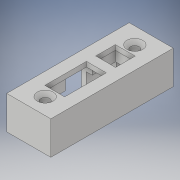
# Autodesk Inventor part: sharp1
Saved by Autodesk Inventor 2019 (Build 230136000, 136)
## iProperties
Created: 2019-04-30
Part Number: sharp1
Material: Générique
Document SubType Name: Modeling
Designer: dubicube
Density: 1 g/cm^3
Appearance: Par défaut
Author: dubicube
Autodesk Inventor part; units mm, degrees
ref_plane "YZ Plane" through (0, 0, 0) normal (1, 0, 0) x (0, 1, 0)
ref_plane "XZ Plane" through (0, 0, 0) normal (0, 1, 0) x (-1, 0, 0)
ref_plane "XY Plane" through (0, 0, 0) normal (0, 0, 1) x (1, 0, 0)
sketch "Esquisse1" plane through (0, 0, 0) normal (0, 1, 0) x (-1, 0, 0)
  line L0 (0, 0) -> (-18, 0)
  line L1 (-18, 0) -> (-18, -50)
  line L2 (-18, -50) -> (0, -50)
  line L3 (0, -50) -> (0, 0)
  dimension "d0" = 50
  dimension "d1" = 18
  constraints: 8 end point, 2 parallel, 1 coincident, 1 horizontal, 1 perpendicular
  measures "d0" distance of L2.end L0.start
  measures "d1" distance of L0.start L0.end
extrude "Extrusion1" add sketch "Esquisse1" along normal blind 13.6
sketch "Esquisse2" plane through (0, 0, 0) normal (0, -1, 0) x (1, 0, 0)
  line L0 (13.05, -10.6) -> (4.95, -10.6)
  line L1 (4.95, -10.6) -> (4.95, -27.6)
  line L2 (4.95, -39.4) -> (13.05, -39.4)
  line L3 (13.05, -39.4) -> (13.05, -31.4)
  line L4 (18, 0) -> (18, -50) projected
  line L5 (18, -25) -> (0, -25) construction
  line L6 (0, -50) -> (0, 0) projected
  line L7 (0, 0) -> (18, 0) projected
  line L8 (9, 0) -> (9, -50) construction
  line L9 (18, -50) -> (0, -50) projected
  line L10 (13.05, -31.4) -> (4.95, -31.4)
  line L11 (4.95, -27.6) -> (13.05, -27.6)
  line L12 (13.05, -31.4) -> (13.05, -27.6) construction
  line L13 (13.05, -27.6) -> (13.05, -10.6)
  line L14 (4.95, -27.6) -> (4.95, -31.4) construction
  line L15 (4.95, -31.4) -> (4.95, -39.4)
  point P0 (13.05, -25)
  point P1 (9, -10.6)
  dimension "d4" = 28.8
  dimension "d5" = 8.1
  dimension "d36" = 8
  dimension "d37" = 17
  constraints: 24 end point, 10 parallel, 9 perpendicular, 5 midpoint, 4 point on line, 1 horizontal
  measures "d4" distance of L2.end L0.start
  measures "d5" distance of L0.start L0.end
  measures "d36" distance between parallel lines of L2 L10
  measures "d37" distance between parallel lines of L0 L11
extrude "Extrusion2" cut sketch "Esquisse2" against normal blind 13.6 contours L13 L11 L1 L0 | L15 L10 L3 L2
sketch "Esquisse3" plane through (0, 0, 0) normal (0, -1, 0) x (1, 0, 0)
  circle A0 centre (9, -43.3) radius 1.75
  line L0 (4.95, -10.6) -> (13.05, -10.6) projected
  line L1 (0, -50) -> (0, 0) projected
  line L2 (18, -50) -> (0, -50) projected
  line L3 (9, -50) -> (9, 0)
  line L4 (0, 0) -> (18, 0) projected
  circle A1 centre (9, -6.7) radius 1.75
  line L5 (13.05, -39.4) -> (4.95, -39.4) projected
  dimension "d8" = 32.7
  dimension "d10" = 3.5
  dimension "d11" = 3.5
  dimension "d12" = 32.7
  constraints: 2 centre point, 2 end point, 2 midpoint, 2 point on line
  measures "d8" distance from line of A0.centre L0
  measures "d10" diameter of A0
  measures "d11" diameter of A1
  measures "d12" distance from line of A1.centre L5
extrude "Extrusion3" cut sketch "Esquisse3" against normal blind 13.6 contours A0 L3 | L3 A0 | A1 L3 | L3 A1
sketch "Esquisse4" plane through (0, 0, 0) normal (0, -1, 0) x (1, 0, 0)
  line L0 (13.55, -10) -> (13.55, -40)
  line L1 (13.55, -40) -> (4.45, -40)
  line L2 (4.45, -40) -> (4.45, -30.5)
  line L3 (4.45, -30.5) -> (0, -30.5)
  line L4 (0, -30.5) -> (0, -19.5)
  line L5 (0, -50) -> (0, 0) projected
  line L6 (0, -19.5) -> (4.45, -19.5)
  line L7 (4.45, -19.5) -> (4.45, -10)
  line L8 (4.45, -10) -> (13.55, -10)
  line L9 (18, 0) -> (18, -50) projected
  line L10 (18, -25) -> (0, -25) construction
  line L11 (0, 0) -> (18, 0) projected
  line L12 (9, 0) -> (9, -50) construction
  line L13 (0, -50) -> (0, 0) projected
  point P0 (13.55, -25)
  point P1 (9, -10)
  dimension "d15" = 30
  dimension "d16" = 9.1
  dimension "d17" = 11
  constraints: 20 end point, 7 midpoint, 5 perpendicular, 5 point on line, 2 vertical
  measures "d15" distance of L0.start L0.end
  measures "d16" distance of L0.end L1.end
  measures "d17" distance of L3.end L4.end
extrude "Extrusion4" cut sketch "Esquisse4" against normal blind 11.6
sketch "Esquisse5" plane through (0, 0, 0) normal (0, -1, 0) x (1, 0, 0)
  line L0 (16, -10) -> (16, -40)
  line L1 (16, -40) -> (13.25, -40)
  line L2 (13.25, -40) -> (13.25, -43)
  line L3 (13.25, -43) -> (4.75, -43)
  line L4 (4.75, -43) -> (4.75, -40)
  line L5 (4.75, -40) -> (2, -40)
  line L6 (2, -40) -> (2, -10)
  line L7 (2, -10) -> (4.75, -10)
  line L8 (4.75, -10) -> (4.75, -7)
  line L9 (4.75, -7) -> (13.25, -7)
  line L10 (13.25, -7) -> (13.25, -10)
  line L11 (16, -10) -> (13.25, -10)
  line L12 (0, 0) -> (18, 0) projected
  line L13 (9, 0) -> (9, -50)
  line L14 (18, -50) -> (0, -50) projected
  line L15 (0, -30.5) -> (0, -19.5) projected
  line L16 (0, -25) -> (9, -25)
  line L17 (4.45, -10) -> (13.55, -10) projected
  point P0 (2, -25)
  point P1 (9, -7)
  dimension "d20" = 14
  dimension "d21" = 36
  dimension "d22" = 8.5
  constraints: 28 end point, 9 point on line, 8 perpendicular, 6 midpoint, 3 collinear, 1 vertical
  measures "d20" distance between parallel lines of L6 L0
  measures "d21" distance between parallel lines of L3 L9
  measures "d22" distance of L8.end L9.end
extrude "Extrusion5" cut sketch "Esquisse5" against normal blind 7
sketch "Esquisse6" plane through (0, 0, 0) normal (0, -1, 0) x (1, 0, 0)
  circle A0 centre (9, -6.7) radius 4.25
  arc A1 (10.7241, -7) -> (7.2759, -7) centre (9, -6.7) ccw projected
  circle A2 centre (9, -43.3) radius 4.25
  arc A3 (10.7241, -43) -> (7.2759, -43) centre (9, -43.3) ccw projected
  point P0 (0, 0)
  dimension "d25" = 8.5
  dimension "d26" = 8.5
  constraints: 2 centre point, 2 concentric
  measures "d25" diameter of A0
  measures "d26" diameter of A2
extrude "Extrusion6" cut sketch "Esquisse6" against normal blind 1.5
chamfer "Chanfrein1" distance 1.5 angle 45 1 edges at (7.25, 13.6, -6.7)
chamfer "Chanfrein2" distance 1.5 angle 45 1 edges at (7.25, 13.6, -43.3)
equation "\"d11\" = d10"
equation "\"d12\" = d8"
